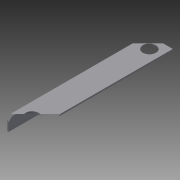
# Autodesk Inventor part: chainguard
Saved by Autodesk Inventor 2016 (Build 200138000, 138)
## iProperties
Created: 2016-01-27
Part Number: chainguard
Material: Generic
Document SubType Name: Modeling
Designer: 278648
Density: 1 g/cm^3
Appearance: Default
Mass: 72.7421 g
Surface Area: 488.314 cm^2
Volume: 72.7421 cm^3
Author: 278648
Autodesk Inventor part; units mm, degrees
ref_plane "YZ Plane" through (0, 0, 0) normal (1, 0, 0) x (0, 1, 0)
ref_plane "XZ Plane" through (0, 0, 0) normal (0, 1, 0) x (-1, 0, 0)
ref_plane "XY Plane" through (0, 0, 0) normal (0, 0, 1) x (1, 0, 0)
sketch "Sketch1" plane through (0, 0, 0) normal (0, 1, 0) x (-1, 0, 0)
  line L0 (0, 0) -> (-50.8, 0)
  line L1 (-50.8, 0) -> (-50.8, -304.8)
  line L2 (-50.8, -304.8) -> (0, -304.8)
  line L3 (0, -304.8) -> (0, 0)
  circle A0 centre (-25.4, -25.4) radius 14.2875
  circle A1 centre (-25.4, -279.4) radius 14.2875
  dimension "d0" = 304.8
  dimension "d1" = 50.8
  dimension "d2" = 25.4
  dimension "d3" = 25.4
  dimension "d4" = 25.4
  dimension "d5" = 25.4
  dimension "d6" = 28.575
  dimension "d7" = 28.575
  constraints: 8 end point, 2 centre point, 2 parallel, 1 horizontal, 1 perpendicular
  measures "d0" distance between parallel lines of L0 L2
  measures "d1" distance between parallel lines of L3 L1
  measures "d2" distance from line of L3 A0.centre
  measures "d3" distance from line of L3 A1.centre
  measures "d4" distance from line of L0 A0.centre
  measures "d5" distance from line of L2 A1.centre
  measures "d6" diameter of A0
  measures "d7" diameter of A1
extrude "Extrusion1" add sketch "Sketch1" along normal blind 3.175
sketch "Sketch2" plane through (0, 0, -304.8) normal (-1, 0, 0) x (0, 0, 1)
  line L0 (304.8, 3.175) -> (0, 3.175)
  line L1 (0, 3.175) -> (0, 0)
  line L2 (0, 0) -> (304.8, 0)
  line L3 (304.8, 0) -> (304.8, 3.175)
  constraints: 8 end point, 2 parallel, 1 horizontal, 1 perpendicular
extrude "Extrusion2" add sketch "Sketch2" along normal blind 3.175
sketch "Sketch3" plane through (0, 0, 0) normal (0, -1, 0) x (1, 0, 0)
  line L0 (0, 0) -> (-3.175, 0)
  line L1 (-3.175, 0) -> (-3.175, -304.8)
  line L2 (-3.175, -304.8) -> (0, -304.8)
  line L3 (0, -304.8) -> (0, 0)
  constraints: 8 end point, 2 parallel, 1 horizontal, 1 perpendicular
extrude "Extrusion3" add sketch "Sketch3" along normal blind 25.4
body "Solid1"
